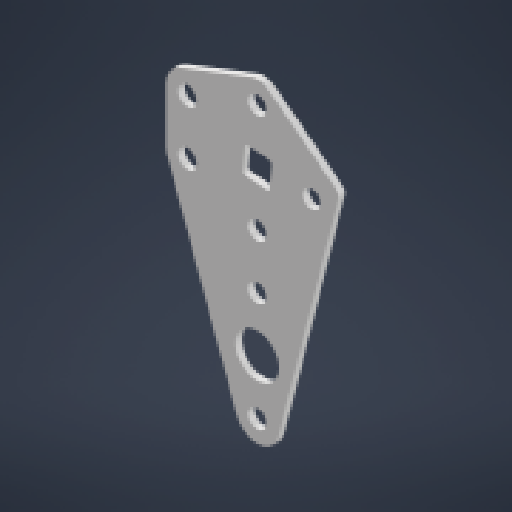
# Autodesk Inventor part: coffin-v2
Saved by Autodesk Inventor 2023.2 (Build 272271000, 271)
## iProperties
Created: 2023-04-01
Part Number: coffin-v2
Material: Generic
Document SubType Name: Modeling
Designer: Liam
Density: 1 g/cm^3
Appearance: Default
Author: Liam
Autodesk Inventor part; units mm, degrees
ref_plane "YZ Plane" through (0, 0, 0) normal (1, 0, 0) x (0, 1, 0)
ref_plane "XZ Plane" through (0, 0, 0) normal (0, 1, 0) x (-1, 0, 0)
ref_plane "XY Plane" through (0, 0, 0) normal (0, 0, 1) x (1, 0, 0)
sketch "Sketch1" plane through (0, 0, 0) normal (0, 0, 1) x (1, 0, 0)
  line L0 (36.3823, 2.8212) -> (22.3659, -52.0571)
  arc A0 (12.6742, -52.5484) -> (22.3659, -52.0571) centre (17.4439, -50.8) ccw
  line L1 (12.6742, -52.5484) -> (-3.6199, -8.0984)
  arc A1 (-3.9302, -6.35) -> (-3.6199, -8.0984) centre (1.1498, -6.35) ccw
  line L2 (-3.9302, -6.35) -> (-3.9302, 6.35)
  arc A2 (-0.6948, 11.0833) -> (-3.9302, 6.35) centre (1.1498, 6.35) ccw
  line L3 (-0.6948, 11.0833) -> (15.5993, 17.4333)
  arc A3 (20.8415, 2.2589) -> (20.2651, 2.9475) centre (20.209, 2.315) ccw
  line L4 (20.2651, 2.9475) -> (15.185, 3.3976)
  arc A4 (15.185, 3.3976) -> (14.4964, 2.8212) centre (15.1289, 2.7651) ccw
  line L5 (14.4964, 2.8212) -> (14.0462, -2.2589)
  arc A5 (14.0462, -2.2589) -> (14.6227, -2.9475) centre (14.6788, -2.315) ccw
  line L6 (14.6227, -2.9475) -> (19.7028, -3.3976)
  arc A6 (19.7028, -3.3976) -> (20.3914, -2.8212) centre (19.7589, -2.7651) ccw
  line L7 (20.3914, -2.8212) -> (20.8415, 2.2589)
  circle A7 centre (17.4439, -38.1) radius 5.08
  circle A8 centre (17.4439, -25.4) radius 2.1082
  circle A9 centre (17.4439, -12.7) radius 2.1082
  circle A10 centre (30.1439, 0) radius 2.1082
  circle A11 centre (17.4439, 12.7) radius 2.1082
  circle A12 centre (1.1498, 6.35) radius 2.1844
  circle A13 centre (1.1498, -6.35) radius 2.1844
  circle A14 centre (17.4439, -50.8) radius 2.0955
  line L8 (21.036, 16.2921) -> (34.5847, 5.9063)
  spline S0 degree 4 poles (15.5993, 17.4333) (16.2989, 17.7059) (17.6982, 18.2512) (19.3014, 17.6218) (20.4578, 16.7353) (21.036, 16.2921) knots 0 0 0 0 0 0.5 1 1 1 1 1
  line L9 (15.5993, 17.4333) -> (16.2989, 17.7059) construction
  line L10 (16.2989, 17.7059) -> (17.6982, 18.2512) construction
  line L11 (17.6982, 18.2512) -> (19.3014, 17.6218) construction
  line L12 (19.3014, 17.6218) -> (20.4578, 16.7353) construction
  line L13 (20.4578, 16.7353) -> (21.036, 16.2921) construction
  spline S1 degree 4 poles (34.5847, 5.9063) (34.9521, 5.6246) (35.6871, 5.0612) (36.7613, 4.305) (36.5086, 3.3158) (36.3823, 2.8212) knots 0 0 0 0 0 0.5 1 1 1 1 1
  point P0 (-3.9302, 6.35)
  point P1 (-3.9302, -6.35)
  point P2 (-3.6199, -8.0984)
  point P3 (12.6742, -52.5484)
  point P4 (21.7462, -53.5011)
  point P5 (21.0356, 16.2924)
  point P6 (15.5996, 17.4334)
  point P7 (20.8415, 2.2589)
  point P8 (20.3914, -2.8212)
  point P9 (14.6227, -2.9475)
  point P10 (14.4964, 2.8212)
  point P11 (20.2651, 2.9475)
  dimension "d0" = 4.3688
  dimension "d1" = 4.3688
  dimension "d2" = 4.2164
  dimension "d3" = 4.2164
  dimension "d5" = 4.2164
  dimension "d6" = 4.2164
  dimension "d7" = 10.16
  dimension "d8" = 4.191
  constraints: 18 end point, 15 centre point, 14 point on circle, 1 tangent, 32 other
  measures "d0" diameter of A12
  measures "d1" diameter of A13
  measures "d2" diameter of A11
  measures "d3" diameter of A10
  measures "d5" diameter of A9
  measures "d6" diameter of A8
  measures "d7" diameter of A7
  measures "d8" diameter of A14
extrude "Extrusion1" add sketch "Sketch1" along normal blind 1.524
body "Solid1"
